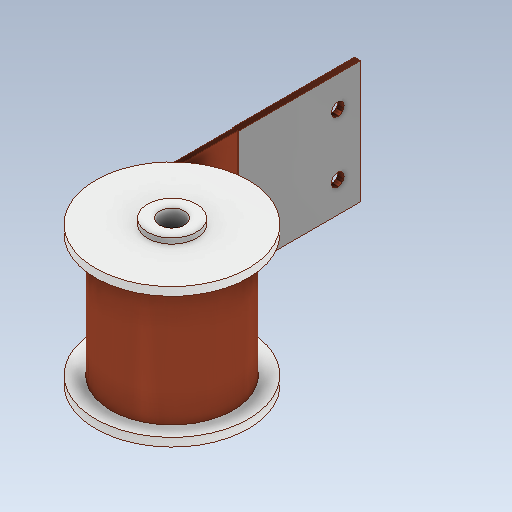
# Autodesk Inventor part: 定荷重バネ49N
Saved by Autodesk Inventor 2020 (Build 240168000, 168)
## iProperties
Created: 2020-01-16
Part Number: 定荷重バネ49N
Material: アルミニウム 6061
Document SubType Name: Modeling
Designer: yuta2
Density: 3.25674 g/cm^3
Appearance: 銅 - つや出し
Mass: 210 g
Surface Area: 186.322 cm^2
Volume: 64.4817 cm^3
Author: yuta2
Autodesk Inventor part; units mm, degrees
ref_plane "YZ Plane" through (0, 0, 0) normal (1, 0, 0) x (0, 1, 0)
ref_plane "XZ Plane" through (0, 0, 0) normal (0, 1, 0) x (-1, 0, 0)
ref_plane "XY Plane" through (0, 0, 0) normal (0, 0, 1) x (1, 0, 0)
sketch "スケッチ1" plane through (0, 0, 0) normal (1, 0, 0) x (0, 1, 0)
  line L0 (0, 0) -> (2.75, 0)
  line L1 (2.75, 0) -> (2.75, -25)
  line L2 (2.75, -25) -> (0, -25)
  line L3 (0, -25) -> (0, 0)
  line L4 (2.75, 0) -> (42.75, 0)
  line L5 (42.75, 0) -> (42.75, -20)
  line L6 (42.75, -20) -> (2.75, -20)
  line L7 (2.75, -20) -> (2.75, 0)
  line L8 (42.75, 0) -> (45.5, 0)
  line L9 (45.5, 0) -> (45.5, -25)
  line L10 (45.5, -25) -> (42.75, -25)
  line L11 (42.75, -25) -> (42.75, 0)
  line L12 (22.75, 0) -> (22.75, -20)
  line L13 (45.5, 0) -> (47.25, 0)
  line L14 (47.25, 0) -> (47.25, -8)
  line L15 (47.25, -8) -> (45.5, -8)
  line L16 (45.5, -8) -> (45.5, 0)
  line L17 (0, 0) -> (-1.75, 0)
  line L18 (-1.75, 0) -> (-1.75, -8)
  line L19 (-1.75, -8) -> (0, -8)
  line L20 (0, -8) -> (0, 0)
  line L21 (47.25, 0) -> (-1.75, 0)
  line L22 (-1.75, 0) -> (-1.75, -4.05)
  line L23 (-1.75, -4.05) -> (47.25, -4.05)
  line L24 (47.25, -4.05) -> (47.25, 0)
  point P0 (2.75, -20)
  point P1 (42.75, -20)
  dimension "d0" = 45.5
  dimension "d1" = 25
  dimension "d2" = 20
  dimension "d3" = 49
  dimension "d4" = 8
  dimension "d5" = 4.05
  dimension "d11" = 40
  constraints: 50 end point, 12 parallel, 6 horizontal, 6 perpendicular, 2 midpoint, 1 horizontal alignment, 1 point on line, 3 other
  measures "d0" distance between parallel lines of L3 L9
  measures "d1" distance between parallel lines of L10 L4
  measures "d2" distance between parallel lines of L4 L6
  measures "d3" distance between parallel lines of L18 L14
  measures "d4" distance between parallel lines of L8 L15
  measures "d5" distance of L22.end L21.end
  measures "d11" distance between parallel lines of L7 L5
revolve "回転1" add sketch "スケッチ1" angle 360 about axis through (0, 2.75, 0) along (0, 1, 0) contours L23 L1 L2 L3 | L3 L19 L18 L23 | L23 L12 L6 L1 | L23 L5 L6 L12 | L23 L9 L10 L11 L5 | L23 L14 L15 L9
sketch "スケッチ2" plane through (0, 2.75, 0) normal (0, 1, 0) x (1, 0, 0)
  circle A0 centre (0, 0) radius 20 projected
  line L0 (-20, 0) -> (-20, 80)
  line L1 (-20, 80) -> (-18.5, 80)
  line L2 (-18.5, 80) -> (-18.5, 7.5993)
  circle A1 centre (0, 0) radius 20
  point P0 (0, 0)
  dimension "d7" = 80
  dimension "d8" = 1.5
  constraints: 6 end point, 2 point on circle, 1 centre point, 1 coincident, 1 concentric, 1 parallel, 1 perpendicular, 1 tangent, 1 vertical
  measures "d7" distance of L0.start L0.end
  measures "d8" distance of L0.end L1.end
extrude "押し出し1" add sketch "スケッチ2" along normal blind 40 contours A0 L0 L1 L2
sketch "スケッチ4" plane through (-20, 2.75, -80) normal (-1, 0, 0) x (0, 0, 1)
  line L0 (0, 40) -> (65, 40) projected
  line L1 (0, 40) -> (40, 40)
  line L2 (40, 40) -> (40, 0)
  line L3 (40, 0) -> (0, 0)
  line L4 (0, 0) -> (0, 40)
  point P0 (80, -2.75)
  dimension "d12" = 40
  dimension "d13" = 40
  constraints: 8 end point, 2 parallel, 1 horizontal, 1 perpendicular
  measures "d12" distance of L2.end L3.end
  measures "d13" distance of L1.end L2.end
extrude "押し出し2" add sketch "スケッチ4" along normal blind 0.25
sketch "スケッチ5" plane through (-18.5, 2.75, -16.8152) normal (1, 0, 0) x (0, 0, -1)
  line L0 (63.1848, 0) -> (63.1848, 40) projected
  line L1 (0, 0) -> (63.1848, 0) projected
  line L2 (63.1848, 40) -> (23.1848, 40)
  line L3 (23.1848, 40) -> (23.1848, 0)
  line L4 (23.1848, 0) -> (63.1848, 0)
  line L5 (63.1848, 0) -> (63.1848, 40)
  point P0 (-16.8152, -2.75)
  dimension "d16" = 40
  constraints: 8 end point, 2 parallel, 1 horizontal, 1 perpendicular, 1 point on line
  measures "d16" distance of L4.end L3.end
extrude "押し出し3" add sketch "スケッチ5" along normal blind 0.25
sketch "スケッチ6" plane through (-18.25, 2.75, -16.8152) normal (1, 0, 0) x (0, 0, -1)
  line L0 (63.1848, 40) -> (63.1848, 0) projected
  line L1 (63.1848, 20) -> (23.1848, 20)
  line L2 (23.1848, 0) -> (23.1848, 40) projected
  point P0 (-16.8152, -2.75)
  point P1 (55.6848, 30)
  point P2 (55.6848, 10)
  dimension "d19" = 20
  dimension "d20" = 7.5
  constraints: 2 end point, 2 midpoint, 1 symmetric about line
  measures "d19" distance of point (55.685, 10) point (55.685, 30)
  measures "d20" distance from line of L0 point (55.685, 30)
hole "穴1" at (-18.25, 32.75, -72.5) at (-18.25, 12.75, -72.5) direction (-1, 0, 0) diameter 4.2 end through all
equation "\"d1\" = 0.5 * SpringD"
equation "\"d3\" = SpringWidth"
equation "\"SpringD\" = 50"
equation "\"SpringWidth\" = 49"
